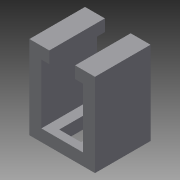
# Autodesk Inventor part: SoporteVentosa
Saved by Autodesk Inventor 2014 SP1 (Build 180222100, 222)
## iProperties
Created: 2014-03-18
Part Number: SoporteVentosa
Material: Genérico
Document SubType Name: Modeling
Designer: Gregorio
Density: 1 g/cm^3
Appearance: Valor por defecto
Author: Gregorio
Autodesk Inventor part; units mm, degrees
ref_plane "YZ Plane" through (0, 0, 0) normal (1, 0, 0) x (0, 1, 0)
ref_plane "XZ Plane" through (0, 0, 0) normal (0, 1, 0) x (-1, 0, 0)
ref_plane "XY Plane" through (0, 0, 0) normal (0, 0, 1) x (1, 0, 0)
sketch "Boceto1" plane through (0, 0, 0) normal (0, 1, 0) x (-1, 0, 0)
  line L0 (0, 0) -> (3, 0)
  line L1 (3, 0) -> (3, 18)
  line L2 (3, 18) -> (0, 18)
  line L3 (0, 18) -> (0, 0)
  line L4 (0, 0) -> (16.5, 0)
  line L5 (16.5, 0) -> (16.5, 3)
  line L6 (16.5, 3) -> (0, 3)
  line L7 (0, 3) -> (0, 0)
  line L8 (16.5, 0) -> (13.5, 0)
  line L9 (13.5, 0) -> (13.5, 18)
  line L10 (13.5, 18) -> (16.5, 18)
  line L11 (16.5, 18) -> (16.5, 0)
  line L12 (0, 18) -> (5, 18)
  line L13 (5, 18) -> (5, 21)
  line L14 (5, 21) -> (0, 21)
  line L15 (0, 21) -> (0, 18)
  line L16 (16.5, 18) -> (11.5, 18)
  line L17 (11.5, 18) -> (11.5, 21)
  line L18 (11.5, 21) -> (16.5, 21)
  line L19 (16.5, 21) -> (16.5, 18)
  dimension "d0" = 3
  dimension "d1" = 18
  dimension "d2" = 16.5
  dimension "d3" = 3
  dimension "d4" = 18
  dimension "d5" = 5
  dimension "d6" = 5
  dimension "d14" = 3
  dimension "d15" = 3
  constraints: 40 end point, 10 parallel, 5 horizontal, 5 perpendicular
  measures "d0" distance of L2.end L1.end
  measures "d1" distance of L1.end L0.end
  measures "d2" distance of L6.end L5.end
  measures "d3" distance of L9.end L10.end
  measures "d4" distance of L10.end L4.end
  measures "d5" distance of L13.end L14.end
  measures "d6" distance of L17.end L18.end
  measures "d14" distance of L18.end L10.end
  measures "d15" distance of L14.end L2.end
extrude "Extrusión1" add sketch "Boceto1" along normal blind 14
sketch "Boceto3" plane through (0, 0, 0) normal (0, 0, -1) x (-1, 0, 0)
  line L0 (11, 2) -> (5.5, 2)
  line L1 (5.5, 2) -> (5.5, 12)
  line L2 (5.5, 12) -> (11, 12)
  line L3 (11, 12) -> (11, 2)
  line L4 (11, 2) -> (5.5, 12) construction
  line L5 (5.5, 2) -> (11, 12) construction
  point P0 (8.25, 7)
  dimension "d10" = 5.5
  dimension "d11" = 10
  constraints: 12 end point, 2 midpoint, 2 parallel, 1 horizontal, 1 perpendicular
  measures "d10" distance of L1.end L2.end
  measures "d11" distance of L0.end L1.end
extrude "Extrusión2" cut sketch "Boceto3" against normal blind 10
